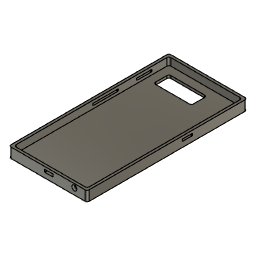
OnePlus 5 deksel (Autodesk Fusion 360 design; units mm, degrees)
Autodesk Fusion 360 part; units mm, degrees
sketch "Sketch1" plane through (0, 0, 0) normal (0, 0, 1) x (1, 0, 0)
  line L0 (0, 0) -> (76.6, 0)
  line L1 (76.6, 0) -> (76.6, 156.7)
  line L2 (76.6, 156.7) -> (0, 156.7)
  line L3 (0, 156.7) -> (0, 0)
  dimension "d5" = 76.6
  dimension "d6" = 156.7
  constraint horizontal L0
  constraint vertical L1
  constraint horizontal L2
  constraint vertical L3
  constraint coincident L0.start L3.end
  measures "d5" distance of L0.start L0.end
  measures "d6" distance of L0.start L2.end
extrude "Extrude1" add sketch "Sketch1" along normal blind 2.5
sketch "Sketch2" plane through (0, 0, 2.5) normal (0, 0, 1) x (-1, 0, 0)
  line L0 (0, -156.7) -> (0, 0)
  line L1 (0, 0) -> (-76.6, 0)
  line L2 (-76.6, 0) -> (-76.6, -156.7)
  line L3 (-76.6, -156.7) -> (0, -156.7)
  line L4 (-2.5, -154.2) -> (-74.1, -154.2)
  line L5 (-74.1, -154.2) -> (-74.1, -2.5)
  line L6 (-74.1, -2.5) -> (-2.5, -2.5)
  line L7 (-2.5, -2.5) -> (-2.5, -154.2)
  dimension "d13" = 2.5
  dimension "d14" = 2.5
  dimension "d15" = 2.5
  dimension "d16" = 2.5
  constraint horizontal L4
  constraint vertical L5
  constraint horizontal L6
  constraint vertical L7
  measures "d13" distance of L2 L5
  measures "d14" distance of L0 L7
  measures "d15" distance of L3 L4
  measures "d16" distance of L1 L6
extrude "Extrude2" add sketch "Sketch2" along normal blind 7.25
fillet "Fillet1" radius 2 4 edges at (74.1, 154.2, 6.125) (2.5, 154.2, 6.125) (74.1, 2.5, 6.125) (2.5, 2.5, 6.125)
fillet "Fillet2" radius 2 4 edges at (0, 0, 4.875) (0, 156.7, 4.875) (76.6, 0, 4.875) (76.6, 156.7, 4.875)
sketch "Sketch3" plane through (0, 0, 2.5) normal (0, 0, 1) x (-1, 0, 0)
  arc A0 (-2.5, -4.5) -> (-4.5, -2.5) centre (-4.5, -4.5) ccw
  line L0 (-4.5, -2.5) -> (-72.1, -2.5)
  arc A1 (-72.1, -2.5) -> (-74.1, -4.5) centre (-72.1, -4.5) ccw
  line L1 (-74.1, -4.5) -> (-74.1, -152.2)
  arc A2 (-74.1, -152.2) -> (-72.1, -154.2) centre (-72.1, -152.2) ccw
  line L2 (-72.1, -154.2) -> (-4.5, -154.2)
  arc A3 (-4.5, -154.2) -> (-2.5, -152.2) centre (-4.5, -152.2) ccw
  line L3 (-2.5, -152.2) -> (-2.5, -4.5)
  line L4 (-10.5, -146.2) -> (-47.55, -146.2)
  line L5 (-47.55, -146.2) -> (-47.55, -131.2)
  line L6 (-47.55, -131.2) -> (-10.5, -131.2)
  line L7 (-10.5, -131.2) -> (-10.5, -146.2)
  dimension "d28" = 37.05
  dimension "d29" = 15
  dimension "d30" = 37.05
  dimension "d31" = 8
  dimension "d32" = 8
  constraint horizontal L4
  constraint vertical L5
  constraint horizontal L6
  constraint vertical L7
  measures "d28" distance of L4.start L4.end
  measures "d29" distance of L4.start L6.end
  measures "d30" distance of L4.start L4.end
  measures "d31" distance of L3 L7
  measures "d32" distance of L2 L4
extrude "Extrude3" cut sketch "Sketch3" against normal blind 10 contours L4 L5 L6 L7
fillet "Fillet3" radius 2 4 edges at (10.5, 146.2, 1.25) (47.55, 146.2, 1.25) (47.55, 131.2, 1.25) (10.5, 131.2, 1.25)
sketch "Sketch4" plane through (0, 0, 0) normal (0, -1, 0) x (1, 0, 0)
  line L0 (74.6, 0) -> (74.6, 9.75)
  line L1 (74.6, 9.75) -> (2, 9.75)
  line L2 (2, 9.75) -> (2, 0)
  line L3 (2, 0) -> (74.6, 0)
  line L4 (34.88, 7.405) -> (43.22, 7.405)
  line L5 (43.22, 7.405) -> (43.22, 4.845)
  line L6 (43.22, 4.845) -> (34.88, 4.845)
  line L7 (34.88, 4.845) -> (34.88, 7.405)
  dimension "d39" = 8.34
  dimension "d40" = 2.56
  dimension "d41" = 32.88
  dimension "d42" = 2.345
  constraint horizontal L4
  constraint vertical L5
  constraint horizontal L6
  constraint vertical L7
  measures "d39" distance of L4.start L4.end
  measures "d40" distance of L4.start L6.end
  measures "d41" distance of L2 L7
  measures "d42" distance of L1 L4
extrude "Extrude4" cut sketch "Sketch4" against normal blind 7 contours L4 L5 L6 L7
fillet "Fillet4" radius 0.3 4 edges at (43.22, 1.25, 7.405) (34.88, 1.25, 7.405) (34.88, 1.25, 4.845) (43.22, 1.25, 4.845)
sketch "Sketch5" plane through (0, 0, 0) normal (0, -1, 0) x (1, 0, 0)
  line L0 (43.22, 7.105) -> (43.22, 5.145)
  arc A0 (42.92, 4.845) -> (43.22, 5.145) centre (42.92, 5.145) ccw
  line L1 (42.92, 4.845) -> (35.18, 4.845)
  arc A1 (34.88, 5.145) -> (35.18, 4.845) centre (35.18, 5.145) ccw
  line L2 (34.88, 5.145) -> (34.88, 7.105)
  arc A2 (35.18, 7.405) -> (34.88, 7.105) centre (35.18, 7.105) ccw
  line L3 (35.18, 7.405) -> (42.92, 7.405)
  arc A3 (43.22, 7.105) -> (42.92, 7.405) centre (42.92, 7.105) ccw
  line L4 (74.6, 0) -> (74.6, 9.75)
  line L5 (74.6, 9.75) -> (2, 9.75)
  line L6 (2, 9.75) -> (2, 0)
  line L7 (2, 0) -> (74.6, 0)
  circle A4 centre (64.1, 6.125) radius 2.5
  dimension "d50" = 5
  dimension "d51" = 10.5
  dimension "d52" = 3.625
  measures "d50" diameter of A4
  measures "d51" distance of L4 A4.centre
  measures "d52" distance of L5 A4.centre
extrude "Extrude5" cut sketch "Sketch5" against normal blind 6 contours A4
sketch "Sketch6" plane through (76.6, 0, 0) normal (1, 0, 0) x (0, 1, 0)
  line L0 (154.7, 0) -> (154.7, 9.75)
  line L1 (154.7, 9.75) -> (2, 9.75)
  line L2 (2, 9.75) -> (2, 0)
  line L3 (2, 0) -> (154.7, 0)
  line L4 (93.3, 7.125) -> (103.3, 7.125)
  line L5 (103.3, 7.125) -> (103.3, 5.125)
  line L6 (103.3, 5.125) -> (93.3, 5.125)
  line L7 (93.3, 5.125) -> (93.3, 7.125)
  dimension "d58" = 10
  dimension "d59" = 2
  dimension "d60" = 51.4
  dimension "d61" = 2.625
  constraint horizontal L4
  constraint vertical L5
  constraint horizontal L6
  constraint vertical L7
  measures "d58" distance of L4.start L4.end
  measures "d59" distance of L4.start L6.end
  measures "d60" distance of L0 L5
  measures "d61" distance of L1 L4
extrude "Extrude6" cut sketch "Sketch6" against normal blind 4 contours L4 L5 L6 L7
sketch "Sketch7" plane through (0, 0, 0) normal (-1, 0, 0) x (0, -1, 0)
  line L0 (-154.7, 9.75) -> (-154.7, 0)
  line L1 (-154.7, 0) -> (-2, 0)
  line L2 (-2, 0) -> (-2, 9.75)
  line L3 (-2, 9.75) -> (-154.7, 9.75)
  line L4 (-137.7, 7.125) -> (-122.7, 7.125)
  line L5 (-122.7, 7.125) -> (-122.7, 5.125)
  line L6 (-122.7, 5.125) -> (-137.7, 5.125)
  line L7 (-137.7, 5.125) -> (-137.7, 7.125)
  dimension "d70" = 15
  dimension "d71" = 2
  dimension "d72" = 17
  dimension "d73" = 2.625
  constraint horizontal L4
  constraint vertical L5
  constraint horizontal L6
  constraint vertical L7
  measures "d70" distance of L4.start L4.end
  measures "d71" distance of L4.start L6.end
  measures "d72" distance of L0 L7
  measures "d73" distance of L3 L4
extrude "Extrude7" cut sketch "Sketch7" against normal blind 7 contours L4 L5 L6 L7
sketch "Sketch8" plane through (0, 0, 0) normal (-1, 0, 0) x (0, -1, 0)
  line L0 (-122.7, 7.125) -> (-122.7, 5.125)
  line L1 (-122.7, 5.125) -> (-137.7, 5.125)
  line L2 (-137.7, 5.125) -> (-137.7, 7.125)
  line L3 (-137.7, 7.125) -> (-122.7, 7.125)
  line L4 (-154.7, 9.75) -> (-154.7, 0)
  line L5 (-154.7, 0) -> (-2, 0)
  line L6 (-2, 0) -> (-2, 9.75)
  line L7 (-2, 9.75) -> (-154.7, 9.75)
  line L8 (-104.7, 7.125) -> (-79.7, 7.125)
  line L9 (-79.7, 7.125) -> (-79.7, 5.125)
  line L10 (-79.7, 5.125) -> (-104.7, 5.125)
  line L11 (-104.7, 5.125) -> (-104.7, 7.125)
  dimension "d76" = 25
  dimension "d77" = 2
  dimension "d78" = 18
  dimension "d79" = 2.625
  constraint horizontal L8
  constraint vertical L9
  constraint horizontal L10
  constraint vertical L11
  measures "d76" distance of L8.start L8.end
  measures "d77" distance of L8.start L10.end
  measures "d78" distance of L0 L11
  measures "d79" distance of L7 L8
extrude "Extrude8" cut sketch "Sketch8" against normal blind 5 contours L8 L9 L10 L11
fillet "Fillet5" radius 0.4 4 edges at (1.25, 122.7, 7.125) (1.25, 122.7, 5.125) (1.25, 137.7, 5.125) (1.25, 137.7, 7.125)
fillet "Fillet6" radius 0.4 4 edges at (1.25, 104.7, 7.125) (1.25, 104.7, 5.125) (1.25, 79.7, 7.125) (1.25, 79.7, 5.125)
fillet "Fillet7" radius 0.4 4 edges at (75.35, 93.3, 5.125) (75.35, 103.3, 7.125) (75.35, 103.3, 5.125) (75.35, 93.3, 7.125)
equation "phone_height = 154.2 mm"
equation "phone_width = 74.1 mm"
equation "phone_depth = 7.25 mm"
equation "case_depth = 2.5 mm"
equation "d5 = phone_width + case_depth"
equation "d6 = phone_height + case_depth"
equation "d11 = case_depth"
equation "d13 = case_depth"
equation "d14 = case_depth"
equation "d15 = case_depth"
equation "d16 = case_depth"
equation "d17 = phone_depth"
equation "fillet_amount = 2 mm"
equation "d21 = fillet_amount"
equation "d23 = fillet_amount"
equation "camera_margin_top = 8 mm"
equation "camera_margin_left = 8 mm"
equation "camera_height = 15 mm"
equation "camera_width = phone_width * 0.5"
equation "d28 = camera_width"
equation "d29 = camera_height"
equation "d31 = camera_margin_left"
equation "d32 = camera_margin_top"
equation "d36 = fillet_amount"
equation "usbc_width = 8.34 mm"
equation "usbc_height = 2.56 mm"
equation "d39 = usbc_width"
equation "d40 = usbc_height"
equation "d41 = ( phone_width / 2 ) - ( usbc_width / 2 )"
equation "d42 = ( phone_depth / 2 ) - ( usbc_height / 2 )"
equation "d46 = usb_c_fillet"
equation "usb_c_fillet = 0.3 mm"
equation "aux_diameter = 5 mm"
equation "aux_margin_right = 8 mm"
equation "d50 = aux_diameter"
equation "d51 = aux_margin_right + ( aux_diameter / 2 )"
equation "d52 = phone_depth / 2"
equation "sidebutton_width = 10 mm"
equation "sidebutton_height = 2 mm"
equation "sidebutton_margin_right = phone_height / 3"
equation "d58 = sidebutton_width"
equation "d59 = sidebutton_height"
equation "d60 = sidebutton_margin_right"
equation "d61 = ( phone_depth / 2 ) - ( sidebutton_height / 2 )"
equation "volume_width = 25 mm"
equation "volume_height = 2 mm"
equation "sliderbutton_width = 15 mm"
equation "sliderbutton_height = 2 mm"
equation "sliderbutton_margin_left = 17 mm"
equation "volumebutton_distance_to_sliderbutton = 18 mm"
equation "d70 = sliderbutton_width"
equation "d71 = sliderbutton_height"
equation "d72 = sliderbutton_margin_left"
equation "d73 = ( phone_depth / 2 ) - ( sliderbutton_height / 2 )"
equation "d76 = volume_width"
equation "d77 = volume_height"
equation "d78 = volumebutton_distance_to_sliderbutton"
equation "d79 = ( phone_depth / 2 ) - ( volume_height / 2 )"
equation "button_fillet = 0.4 mm"
equation "d84 = button_fillet"
equation "d86 = button_fillet"
equation "d88 = button_fillet"
